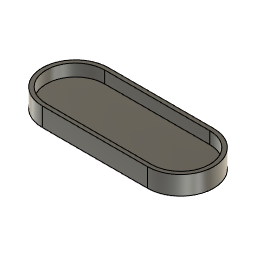
ControllerBaseCOMPONENT_PART (Autodesk Fusion 360 design; units mm, degrees)
Autodesk Fusion 360 part; units mm, degrees
note: some values were not read from the file. Set by a fixed rule: which face or edge a step refers to.
sketch "Base" plane through (0, 0, 0) normal (0, 0, 1) x (1, 0, 0)
  line L0 (0, 0) -> (135, 0)
  line L1 (135, 0) -> (135, -85)
  line L2 (135, -85) -> (0, -85)
  line L3 (0, -85) -> (0, 0)
  arc A0 (0, 0) -> (0, -85) centre (0, -42.5) ccw
  arc A1 (135, -85) -> (135, 0) centre (135, -42.5) ccw
  dimension "d1" = 135
  dimension "d2" = 85
  constraint horizontal L0
  constraint vertical L1
  constraint horizontal L2
  constraint vertical L3
  constraint coincident L0.start L3.end
  constraint tangent L2 A1
  measures "d1" distance of L0.start L0.end
  measures "d2" distance of L0.start L2.end
extrude "Extrude1" add sketch "Base" along normal blind 24
shell "Shell1" thickness 5 removed faces 1 at (45, -56.6667, 24)
extrude "Extrude2" add 1 faces at (90, -55, 5) along direction (0, 0, 1) blind 1.5
extrude "Extrude3" add 1 faces at (90, -55, 6.5) along direction (0, 0, 1) blind 2
named bodies: "BottomPart"
